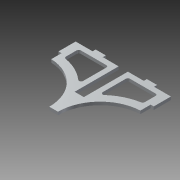
# Autodesk Inventor part: OpenROV 2_3 Dev Ducting Brace
Saved by Autodesk Inventor 2013 (Build 170138000, 138)
## iProperties
Created: 2011-12-01
Part Number: OpenROV 2_3 Dev Ducting Brace
Document SubType Name: Modeling
Designer: user
Density: 1 g/cm^3
Material: Generic
Author: user
Autodesk Inventor part; units mm, degrees
ref_plane "YZ Plane" through (0, 0, 0) normal (1, 0, 0) x (0, 1, 0)
ref_plane "XZ Plane" through (0, 0, 0) normal (0, 1, 0) x (-1, 0, 0)
ref_plane "XY Plane" through (0, 0, 0) normal (0, 0, 1) x (1, 0, 0)
sketch "Sketch1" plane through (0, 0, 0) normal (0, 0, 1) x (1, 0, 0)
  line L0 (-46.5, 0) -> (-46.5, -16.75)
  line L1 (-46.5, -16.75) -> (-43.5, -16.75)
  arc A0 (-4.25, -68) -> (-43.5, -26.7985) centre (-45.5, -68) ccw
  line L2 (-43.5, -16.75) -> (-43.5, -26.7985)
  line L3 (-4.5, 0) -> (-4.5, -43)
  line L4 (-4.5, -43) -> (0, -43)
  line L5 (-20, 0) -> (-20, 3)
  line L6 (-20, 3) -> (-30, 3)
  line L7 (-30, 3) -> (-30, 0)
  line L8 (-46.5, 0) -> (-30, 0)
  line L9 (-20, 0) -> (-4.5, 0)
  line L10 (-38.5, -17.5464) -> (-38.5, -7)
  line L11 (-36.5, -5) -> (-11.5, -5)
  line L12 (-9.5, -7) -> (-9.5, -29.6521)
  arc A1 (-12.8268, -31.1486) -> (-36.8512, -19.5154) centre (-45.5, -68) ccw
  arc A2 (-38.5, -17.5464) -> (-36.8512, -19.5154) centre (-36.5, -17.5464) ccw
  arc A3 (-36.5, -5) -> (-38.5, -7) centre (-36.5, -7) ccw
  arc A4 (-9.5, -7) -> (-11.5, -5) centre (-11.5, -7) ccw
  arc A5 (-12.8268, -31.1486) -> (-9.5, -29.6521) centre (-11.5, -29.6521) ccw
  line L13 (-4.25, -68) -> (0, -68)
  line L14 (46.5, 0) -> (46.5, -16.75)
  line L15 (46.5, -16.75) -> (43.5, -16.75)
  arc A6 (43.5, -26.7985) -> (4.25, -68) centre (45.5, -68) ccw
  line L16 (43.5, -16.75) -> (43.5, -26.7985)
  line L17 (4.5, 0) -> (4.5, -43)
  line L18 (4.5, -43) -> (0, -43)
  line L19 (20, 0) -> (20, 3)
  line L20 (20, 3) -> (30, 3)
  line L21 (30, 3) -> (30, 0)
  line L22 (46.5, 0) -> (30, 0)
  line L23 (20, 0) -> (4.5, 0)
  line L24 (38.5, -17.5464) -> (38.5, -7)
  line L25 (36.5, -5) -> (11.5, -5)
  line L26 (9.5, -7) -> (9.5, -29.6521)
  arc A7 (36.8512, -19.5154) -> (12.8268, -31.1486) centre (45.5, -68) ccw
  arc A8 (36.8512, -19.5154) -> (38.5, -17.5464) centre (36.5, -17.5464) ccw
  arc A9 (38.5, -7) -> (36.5, -5) centre (36.5, -7) ccw
  arc A10 (11.5, -5) -> (9.5, -7) centre (11.5, -7) ccw
  arc A11 (9.5, -29.6521) -> (12.8268, -31.1486) centre (11.5, -29.6521) ccw
  line L27 (4.25, -68) -> (0, -68)
  point P0 (0, 0)
  point P1 (-9.5, -34.391)
  point P2 (-38.5, -19.25)
  point P3 (9.5, -34.391)
  point P4 (38.5, -19.25)
  dimension "d1" = 46.5
  dimension "d3" = 3
  dimension "d5" = 82.5
  dimension "d7" = 45.5
  dimension "d10" = 10
  dimension "d24" = 10
  dimension "d25" = 20
  dimension "d32" = 8
  dimension "d33" = 5
  dimension "d36" = 15.5
  dimension "d37" = 16.5
  dimension "d38" = 16.75
  dimension "d39" = 5
  dimension "d40" = 2
  dimension "d45" = 8
  dimension "d49" = 68
  dimension "d50" = 25
  constraints: 56 end point, 28 point on circle, 12 centre point, 8 tangent, 6 perpendicular, 4 point on line, 3 equal radius, 2 coincident, 2 parallel
  measures "d1" distance of L0.start point (0, 0)
  measures "d3" distance of L0.end L1.end
  measures "d5" diameter of A0
  measures "d7" horizontal distance of point (0, 0) A0.centre
  measures "d10" distance edge to line of A0 L1
  measures "d24" distance of L5.end L6.end
  measures "d25" distance from line of point (0, 0) L5
  measures "d32" distance between parallel lines of L0 L10
  measures "d33" distance between parallel lines of L8 L11
  measures "d36" distance of L5.start L3.start
  measures "d37" distance of L0.start L7.end
  measures "d38" distance of L0.start L0.end
  measures "d39" distance between parallel lines of L3 L12
  measures "d40" radius of A2
  measures "d45" radial gap between concentric circles of A0 A1
  measures "d49" distance between parallel lines of L13 L9
  measures "d50" distance between parallel lines of L13 L4
extrude "Extrusion6" add sketch "Sketch1" along normal blind 3
body "Solid6"
